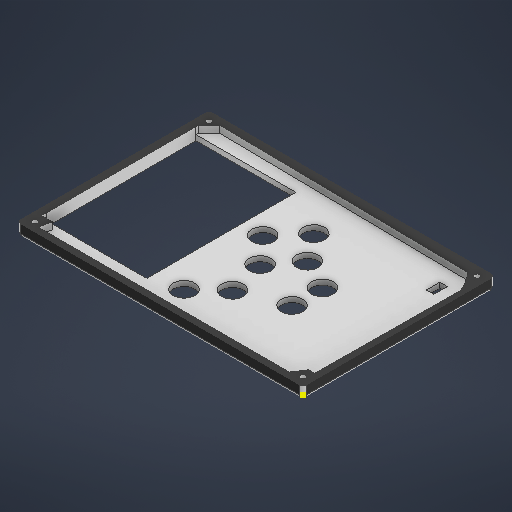
# Autodesk Inventor part: POC
Saved by Autodesk Inventor 2026 (Build 300175050, 175E)
## iProperties
Created: 2025-07-14
Part Number: POC
Material: Generic
Document SubType Name: Modeling
Designer: SaiAn
Density: 1 g/cm^3
Appearance: Default
Author: SaiAn
Autodesk Inventor part; units mm, degrees
ref_plane "YZ Plane" through (0, 0, 0) normal (1, 0, 0) x (0, 1, 0)
ref_plane "XZ Plane" through (0, 0, 0) normal (0, 1, 0) x (-1, 0, 0)
ref_plane "XY Plane" through (0, 0, 0) normal (0, 0, 1) x (1, 0, 0)
sketch "Sketch1" plane through (0, 0, 0) normal (0, 1, 0) x (-1, 0, 0)
  line L0 (0, 0) -> (162.9, 0)
  line L1 (162.9, 0) -> (162.9, -109.326)
  line L2 (162.9, -109.326) -> (0, -109.326)
  line L3 (0, -109.326) -> (0, 0)
  line L4 (152.9, -10) -> (10, -10)
  line L5 (10, -10) -> (10, -99.326)
  line L6 (10, -99.326) -> (152.9, -99.326)
  line L7 (152.9, -99.326) -> (152.9, -10)
  dimension "d0" = 162.9
  dimension "d1" = 109.326
  dimension "d18" = 142.9
  dimension "d19" = 89.326
  dimension "d20" = 10
  dimension "d21" = 10
  constraints: 16 end point, 4 parallel, 2 horizontal, 2 perpendicular
  measures "d0" distance of L1.end L2.end
  measures "d1" distance of L0.end L1.end
  measures "d18" distance of L6.end L5.end
  measures "d19" distance of L5.end L4.end
  measures "d20" distance between parallel lines of L1 L7
  measures "d21" distance between parallel lines of L0 L4
extrude "Extrusion1" add sketch "Sketch1" along normal blind 3 contours L0 L1 L2 L3 | L7 L6 L5 L4
sketch "Sketch2" plane through (0, 3, 0) normal (0, 1, 0) x (1, 0, 0)
  circle A0 centre (-157.9, 5) radius 1.5
  circle A1 centre (-157.9, 104.326) radius 1.5
  circle A2 centre (-5, 5) radius 1.5
  circle A3 centre (-5, 104.326) radius 1.5
  line L0 (-162.9, 0) -> (0, 0) projected
  line L1 (-162.9, 109.326) -> (-162.9, 0) projected
  line L2 (0, 109.326) -> (-162.9, 109.326) projected
  line L3 (0, 0) -> (0, 109.326) projected
  dimension "d4" = 3
  dimension "d5" = 3
  dimension "d6" = 3
  dimension "d7" = 3
  dimension "d8" = 5
  dimension "d9" = 5
  dimension "d10" = 5
  dimension "d11" = 5
  dimension "d12" = 5
  dimension "d13" = 5
  dimension "d14" = 5
  dimension "d15" = 5
  constraints: 4 centre point
  measures "d4" diameter of A0
  measures "d5" diameter of A1
  measures "d6" diameter of A2
  measures "d7" diameter of A3
  measures "d8" distance from line of L0 A0.centre
  measures "d9" distance from line of L1 A0.centre
  measures "d10" distance from line of L1 A1.centre
  measures "d11" distance from line of L2 A1.centre
  measures "d12" distance from line of L3 A2.centre
  measures "d13" distance from line of L0 A2.centre
  measures "d14" distance from line of L3 A3.centre
  measures "d15" distance from line of L2 A3.centre
extrude "Extrusion2" cut sketch "Sketch2" against normal blind 20 contours A0 | A1 | A2 | A3
extrude "Extrusion3" add sketch "Sketch1" along normal blind 7
extrude "Extrusion4" cut sketch "Sketch2" against normal blind 20 contours A0 | A1 | A2 | A3
extrude "Extrusion5" cut sketch "Sketch2" along normal blind 20 contours A0 | A1 | A2 | A3
sketch "Sketch4" plane through (0, 0, 0) normal (0, -1, 0) x (1, 0, 0)
  line L0 (-158.959, -97.964) -> (-102.01, -97.964)
  line L1 (-102.01, -97.964) -> (-102.01, -12.964)
  line L2 (-102.01, -12.964) -> (-158.959, -12.964)
  line L3 (-158.959, -12.964) -> (-158.959, -97.964)
  line L4 (-162.9, -109.326) -> (-162.9, 0) projected
  line L5 (0, -109.326) -> (-162.9, -109.326) projected
  point P0 (0, 0)
  dimension "d34" = 56.949
  dimension "d35" = 85
  dimension "d36" = 3.941
  dimension "d37" = 11.362
  constraints: 8 end point, 2 parallel, 1 horizontal, 1 perpendicular
  measures "d34" distance of L2.end L1.end
  measures "d35" distance of L1.end L0.end
  measures "d36" distance between parallel lines of L4 L3
  measures "d37" distance between parallel lines of L5 L0
extrude "Extrusion7" cut sketch "Sketch4" against normal blind 25
sketch "Sketch5" plane through (0, 7, 0) normal (0, 1, 0) x (1, 0, 0)
  line L0 (-8.1203, 7.8922) -> (-11.1312, 3.3302)
  line L1 (-11.1312, 3.3302) -> (-154.2859, 3.3302)
  line L2 (-154.2859, 3.3302) -> (-152.9, 10)
  line L3 (-152.9, 10) -> (-159.2128, 10)
  line L4 (-158.959, 97.964) -> (-158.959, 12.964) projected
  line L5 (-159.2128, 10) -> (-158.959, 12.964)
  line L6 (-158.959, 12.964) -> (-152.9, 12.964)
  line L7 (-152.9, 12.964) -> (-152.9, 10)
  line L8 (-152.9, 10) -> (-6.7292, 10)
  line L9 (-8.1203, 7.8922) -> (-6.7292, 10)
  line L10 (-152.9, 97.964) -> (-152.9, 99.3125)
  line L11 (-152.9, 99.3125) -> (-159.0859, 99.3125)
  line L12 (-159.0859, 99.3125) -> (-158.959, 97.964)
  line L13 (-158.959, 97.964) -> (-152.9, 97.964)
  line L14 (-159.0859, 99.3125) -> (-152.7487, 105.4257)
  line L15 (-152.7487, 105.4257) -> (-9.2525, 103.4175)
  line L16 (-9.2525, 103.4175) -> (-5.4162, 97.964)
  line L17 (-5.4162, 97.964) -> (-2.61, 92.69)
  line L18 (-2.61, 92.69) -> (-3.2849, 10)
  line L19 (-3.2849, 10) -> (-9.9607, 10)
  line L20 (-9.9607, 10) -> (-9.9607, 99.3125)
  line L21 (-9.9607, 99.3125) -> (-152.9, 99.3125)
  point P0 (0, 0)
  constraints: 42 end point, 7 point on line, 4 perpendicular, 2 parallel, 1 collinear, 1 horizontal, 1 vertical
extrude "Extrusion8" cut sketch "Sketch5" against normal blind 4 contours L0 L1 L2 L8 L9 | L8 L20 L21 L11 L14 L15 L16 L17 L18 L19 | L3 L5 L6 L7 | L10 L13 L12 L11
sketch "Sketch6" plane through (0, 3, 0) normal (0, 1, 0) x (1, 0, 0)
  point P0 (0, 0)
sketch "Sketch7" plane through (-10, 3, -99.3125) normal (-1, 0, 0) x (0, 0, 1)
  line L0 (89.3125, 0) -> (89.3125, 4) projected
  line L1 (0, 0) -> (89.3125, 0)
  line L2 (89.3125, 0) -> (89.3125, 4)
  line L3 (89.3125, 4) -> (0, 4)
  line L4 (0, 4) -> (0, 0)
  point P0 (99.3125, -3)
  constraints: 8 end point, 2 parallel, 1 horizontal, 1 perpendicular
extrude "Extrusion9" cut sketch "Sketch7" against normal blind 0.1
sketch "Sketch8" plane through (0, 0, 0) normal (0, -1, 0) x (1, 0, 0)
  circle A0 centre (-90.1692, -67.2168) radius 6.2
  circle A1 centre (-76.5586, -82.6889) radius 6.2
  circle A2 centre (-64.727, -67.2168) radius 6.2
  circle A3 centre (-76.5586, -52.1169) radius 6.2
  circle A4 centre (-71.7598, -31.5149) radius 6.2
  circle A5 centre (-86.0322, -18.1939) radius 6.2
  circle A6 centre (-47.2771, -58.3169) radius 6.2
  circle A7 centre (-47.2771, -41.0477) radius 6.2
  line L0 (-102.01, -13.9587) -> (-102.01, -97.964)
  line L1 (0, -109.326) -> (-162.9, -109.326) projected
  dimension "d44" = 12.4
  dimension "d45" = 12.4
  dimension "d46" = 12.4
  dimension "d47" = 12.4
  dimension "d48" = 12.4
  dimension "d49" = 12.4
  dimension "d50" = 12.4
  dimension "d51" = 12.4
  constraints: 8 centre point, 2 end point
  measures "d44" diameter of A0
  measures "d45" diameter of A1
  measures "d46" diameter of A2
  measures "d47" diameter of A3
  measures "d48" diameter of A4
  measures "d49" diameter of A5
  measures "d50" diameter of A6
  measures "d51" diameter of A7
extrude "Extrusion10" cut sketch "Sketch8" against normal blind 12.4
sketch "Sketch9" plane through (0, 0, 0) normal (0, -1, 0) x (1, 0, 0)
  line L0 (-16.6242, -94.5996) -> (-12.3494, -94.5996)
  line L1 (-12.3494, -94.5996) -> (-12.3494, -86.9999)
  line L2 (-12.3494, -86.9999) -> (-16.6242, -86.9999)
  line L3 (-16.6242, -86.9999) -> (-16.6242, -94.5996)
  point P0 (0, 0)
  constraints: 8 end point, 2 parallel, 1 horizontal, 1 perpendicular
extrude "Extrusion11" cut sketch "Sketch9" against normal blind 10
sketch "Sketch10" plane through (0, 0, 0) normal (0, -1, 0) x (1, 0, 0)
  arc A0 (-12.0019, -42.7667) -> (-11.8567, -70.2863) centre (-6.0234, -56.4954) ccw construction
  arc A1 (-14.4639, -37.1131) -> (-14.2589, -75.9656) centre (-6.0234, -56.4954) ccw
  arc A2 (-9.5399, -48.4204) -> (-9.4545, -64.607) centre (-6.0234, -56.4954) ccw
  arc A3 (-9.5399, -48.4204) -> (-14.4639, -37.1131) centre (-12.0019, -42.7667) ccw
  arc A4 (-14.2589, -75.9656) -> (-9.4545, -64.607) centre (-11.8567, -70.2863) ccw
  arc A5 (-34.2759, -95.155) -> (-59.3082, -94.0987) centre (-46.8686, -96.4411) ccw construction
  arc A6 (-30.9468, -94.815) -> (-62.5968, -93.4794) centre (-46.8686, -96.4411) ccw
  arc A7 (-37.6051, -95.495) -> (-56.0195, -94.7179) centre (-46.8686, -96.4411) ccw
  arc A8 (-37.6051, -95.495) -> (-30.9468, -94.815) centre (-34.2759, -95.155) ccw
  arc A9 (-62.5968, -93.4794) -> (-56.0195, -94.7179) centre (-59.3082, -94.0987) ccw
  arc A10 (-37.6051, -19.9154) -> (-46.8686, -16.5364) centre (-41.5429, -16.3236) ccw construction
  arc A11 (-36.1848, -21.2109) -> (-48.7894, -16.6132) centre (-41.5429, -16.3236) ccw
  arc A12 (-39.0254, -18.6199) -> (-44.9478, -16.4596) centre (-41.5429, -16.3236) ccw
  arc A13 (-39.0254, -18.6199) -> (-36.1848, -21.2109) centre (-37.6051, -19.9154) ccw
  arc A14 (-48.7894, -16.6132) -> (-44.9478, -16.4596) centre (-46.8686, -16.5364) ccw
  point P0 (0, 0)
  constraints: 30 point on circle, 15 centre point, 12 tangent
extrude "Extrusion12" cut sketch "Sketch10" against normal blind 0.2
fillet "Fillet1" radius 2 4 edges at (-81.45, 0, -109.326) (-81.45, 0, 0) (0, 0, -54.663) (-162.9, 0, -54.663)
fillet "Fillet2" radius 2 8 edges at (0, 4.5, 0) (-0.5858, 0.5858, -0.5858) (-0.5858, 0.5858, -108.7402) (0, 4.5, -109.326) (-162.3142, 0.5858, -0.5858) (-162.9, 4.5, 0) (-162.9, 4.5, -109.326) (-162.3142, 0.5858, -108.7402)
equation "\"d54\" = d50"
body "Solid1"
